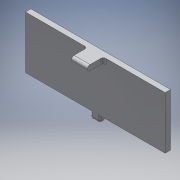
# Autodesk Inventor part: FloppyCover
Saved by Autodesk Inventor 2018 (Build 220112000, 112)
## iProperties
Created: 2019-05-03
Part Number: FloppyCover
Material: PC/ABS Plastic
Document SubType Name: Modeling
Designer: thatg
Density: 0.357273 g/cm^3
Appearance: Smooth - White
Author: thatg
Autodesk Inventor part; units mm, degrees
ref_plane "YZ Plane" through (0, 0, 0) normal (1, 0, 0) x (0, 1, 0)
ref_plane "XZ Plane" through (0, 0, 0) normal (0, 1, 0) x (-1, 0, 0)
ref_plane "XY Plane" through (0, 0, 0) normal (0, 0, 1) x (1, 0, 0)
sketch "Sketch1" plane through (0, 0, 0) normal (0, 0, 1) x (1, 0, 0)
  line L0 (-106.045, 6.985) -> (-90.7112, 6.985) projected
  line L1 (-88.1712, 6.985) -> (-72.8375, 6.985) projected
  line L2 (-72.8375, 6.985) -> (-72.8375, 19.492) projected
  line L3 (-106.045, 19.492) -> (-106.045, 6.985) projected
  line L4 (-106.045, 19.492) -> (-72.8375, 19.492)
  line L5 (-90.0762, 5.207) -> (-88.8062, 5.207)
  line L6 (-88.1712, 6.985) -> (-88.1712, 5.842)
  line L7 (-90.7112, 6.985) -> (-90.7112, 5.842)
  arc A0 (-90.7112, 5.842) -> (-90.0762, 5.207) centre (-90.0762, 5.842) ccw
  arc A1 (-88.8062, 5.207) -> (-88.1712, 5.842) centre (-88.8062, 5.842) ccw
  point P0 (0, 0)
  dimension "d0" = 0.635
  constraints: 8 end point, 4 point on circle, 4 tangent, 2 centre point, 1 equal radius, 1 parallel, 1 perpendicular, 1 vertical
  measures "d0" radius of A0
extrude "Extrusion1" add sketch "Sketch1" along normal blind 1.27
fillet "Fillet1" radius 0.635 10 edges at (-88.3572, 5.393, 0) (-89.4412, 5.207, 0) (-90.5253, 5.393, 0) (-90.7112, 6.4135, 0) (-88.1712, 6.4135, 0) (-88.3572, 5.393, 1.27) (-89.4412, 5.207, 1.27) (-90.5253, 5.393, 1.27) (-90.7112, 6.4135, 1.27) (-88.1712, 6.4135, 1.27)
sketch "Sketch2" plane through (0, 0, 1.27) normal (0, 0, 1) x (1, 0, 0)
  line L0 (-72.8375, 19.492) -> (-106.045, 19.492) projected
  line L1 (-72.8375, 19.492) -> (-106.045, 19.492) projected
  line L2 (-89.4412, 19.492) -> (-89.4412, 18.222)
  line L3 (-89.4412, 18.222) -> (-91.3462, 18.222)
  line L4 (-91.3462, 18.222) -> (-91.3462, 19.492)
  line L5 (-89.4412, 18.222) -> (-87.5362, 18.222)
  line L6 (-87.5362, 18.222) -> (-87.5362, 19.492)
  line L7 (-91.3462, 19.492) -> (-87.5362, 19.492)
  point P0 (0, 0)
  dimension "d4" = 1.27
  dimension "d5" = 1.905
  dimension "d6" = 1.905
  constraints: 12 end point, 3 perpendicular, 3 point on line, 1 collinear, 1 midpoint, 1 vertical
  measures "d4" distance of L2.start L2.end
  measures "d5" distance of L2.end L3.end
  measures "d6" distance of L2.end L5.end
extrude "Extrusion2" add sketch "Sketch2" along normal blind 3.81
fillet "Fillet2" radius 0.635 4 edges at (-89.4412, 19.492, 5.08) (-89.4412, 18.222, 5.08) (-87.5362, 18.857, 1.27) (-91.3462, 18.857, 1.27)
body "Solid1"
